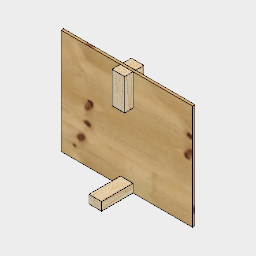
Structural Panel 84 Foot Alanna v1 (Autodesk Fusion 360 design; units mm, degrees)
Autodesk Fusion 360 part; units mm, degrees
box "BoxPrimitive1" add length 40 width 60 height 150 placed x (0, 0, 1) y (1, 0, 0) z (0, 1, 0) at (0, 0, 0) makes body 1
copy_body "Body->Comp1" bodies 1 removing the originals makes body 2 in component "KVH 40x60x150"
box "BoxPrimitive1'" add length 500 width 625 height -12 placed x (0, 1, 0) y (-1, 0, 0) z (0, 0, 1) at (625, 0, 0) separate body makes body 3 in component "PLY 12x500x620"
component "KVH 40x60x150" placed x (1, 0, 0) y (0, 0, 1) z (0, -1, 0) at (0, 40, 0)
component "KVH 40x60x150" placed x (1, 0, 0) y (0, 1, 0) z (0, 0, 1) at (0, 350, 0)
component "PLY 12x500x620" placed x (1, 0, 0) y (0, 1, 0) z (0, 0, 1) at (-282.5, 0, 0)
component "KVH 40x60x150" placed x (1, 0, 0) y (0, 1, 0) z (0, 0, 1) at (0, 350, -52)
component "KVH 40x60x150" placed x (1, 0, 0) y (0, 0, 1) z (0, -1, 0) at (0, 40, -162)
